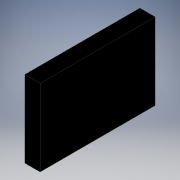
# Autodesk Inventor part: banperparts2
Saved by Autodesk Inventor 2018 (Build 220112000, 112)
## iProperties
Created: 2019-06-17
Part Number: banperparts2
Material: 一般
Document SubType Name: Modeling
Designer: Eiji Nishizawa
Density: 1 g/cm^3
Appearance: 陽極酸化 - 黒
Author: Eiji Nishizawa
Autodesk Inventor part; units mm, degrees
ref_plane "YZ Plane" through (0, 0, 0) normal (1, 0, 0) x (0, 1, 0)
ref_plane "XZ Plane" through (0, 0, 0) normal (0, 1, 0) x (-1, 0, 0)
ref_plane "XY Plane" through (0, 0, 0) normal (0, 0, 1) x (1, 0, 0)
sketch "スケッチ1" plane through (0, 0, 0) normal (1, 0, 0) x (0, 1, 0)
  line L0 (15, 10.4724) -> (0, 10.4724)
  line L1 (0, 10.4724) -> (0, 0.4724)
  line L2 (0, 0.4724) -> (15, 0.4724)
  line L3 (15, 0.4724) -> (15, 10.4724)
  point P0 (0, 0)
  dimension "d0" = 10
  dimension "d1" = 15
  constraints: 8 end point, 2 parallel, 1 horizontal, 1 perpendicular
  measures "d0" distance between parallel lines of L2 L0
  measures "d1" distance of L0.start L0.end
extrude "押し出し1" add sketch "スケッチ1" along normal blind 2
